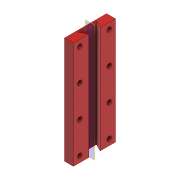
# Autodesk Inventor part: Coupler receiver
Saved by Autodesk Inventor 2020 (Build 240168000, 168)
## iProperties
Created: 2019-11-10
Part Number: Coupler receiver
Material: Generic
Document SubType Name: Modeling
Designer: ball
Density: 1 g/cm^3
Appearance: Default
Author: ball
Autodesk Inventor part; units mm, degrees
ref_plane "YZ Plane" through (0, 0, 0) normal (1, 0, 0) x (0, 1, 0)
ref_plane "XZ Plane" through (0, 0, 0) normal (0, 1, 0) x (-1, 0, 0)
ref_plane "XY Plane" through (0, 0, 0) normal (0, 0, 1) x (1, 0, 0)
sketch "Sketch1" plane through (0, 0, 0) normal (0, 1, 0) x (-1, 0, 0)
  line L0 (0, 17.5) -> (7.366, 17.5)
  line L1 (7.366, 17.5) -> (7.366, -17.5)
  line L2 (7.366, -17.5) -> (0, -17.5)
  line L3 (6.096, 4.754) -> (6.096, -4.754)
  line L4 (0, 4.754) -> (0, 7.802)
  line L5 (6.096, 7.802) -> (6.096, 4.754)
  line L6 (0, -4.754) -> (0, -5.048)
  line L7 (6.096, -7.802) -> (6.096, -4.754)
  line L8 (6.096, 7.802) -> (0, 4.754)
  line L9 (6.096, -7.802) -> (0, -4.754)
  line L10 (0, -17.5) -> (0, -4.754)
  line L11 (0, 4.754) -> (0, 17.5)
  point P0 (0, 0)
  dimension "d0" = 7.366
  dimension "d1" = 35
  dimension "d2" = 17.5
  dimension "d8" = 9.508
  dimension "d9" = 4.754
  dimension "d10" = 3.048
  dimension "d11" = 3.048
  dimension "d12" = 6.096
  dimension "d16" = 15.604
  constraints: 24 end point, 5 parallel, 2 point on line, 1 horizontal, 1 perpendicular
  measures "d0" distance of L1.end L2.end
  measures "d1" distance of L0.end L1.end
  measures "d2" distance from line of L0 point (0, 0)
  measures "d8" distance of L6.start L4.start
  measures "d9" distance of point (0, 0) L4.start
  measures "d10" vertical distance of L5.start L4.start
  measures "d11" vertical distance of L7.start L6.start
  measures "d12" distance from line of L10 L7.start
  measures "d16" distance of L5.start L7.start
extrude "Shape" add sketch "Sketch1" along normal blind 88.9
sketch "Sketch2" plane through (0, 0, -4.754) normal (1, 0, 0) x (0, 0, -1)
  circle A0 centre (7.5184, 5.08) radius 1.9304
  line L0 (3.048, 0) -> (3.048, 88.9) construction
  line L1 (-12.556, 0) -> (-12.556, 88.9) construction
  line L2 (0, 0) -> (12.746, 0) construction
  line L3 (0, 88.9) -> (12.746, 88.9) construction
  circle A1 centre (7.5184, 31.3267) radius 1.9304
  circle A2 centre (7.5184, 57.5733) radius 1.9304
  circle A3 centre (7.5184, 83.82) radius 1.9304
  circle A4 centre (-17.0264, 5.08) radius 1.9304
  line L4 (-22.254, 0) -> (-9.508, 0) construction
  circle A5 centre (-17.0264, 31.3267) radius 1.9304
  circle A6 centre (-17.0264, 57.5733) radius 1.9304
  circle A7 centre (-17.0264, 83.82) radius 1.9304
  point P0 (-4.754, 0)
  dimension "d19" = 3.8608
  dimension "d20" = 4.4704
  dimension "d21" = 88.9
  dimension "d22" = 5.08
  dimension "d25" = 26.2467
  dimension "d30" = 3.8608
  dimension "d31" = 4.4704
  dimension "d32" = 5.08
  dimension "d35" = 26.2467
  constraints: 8 centre point, 2 vertical, 12 other
  measures "d19" diameter of A0
  measures "d20" distance from line of L0 A0.centre
  measures "d21" distance between parallel lines of L2 L3
  measures "d22" distance from line of L2 A0.centre
  measures "d25" distance of A0.centre A1.centre
  measures "d30" diameter of A4
  measures "d31" distance from line of A4.centre L1
  measures "d32" distance from line of L4 A4.centre
  measures "d35" distance of A4.centre A5.centre
extrude "Extrusion2" cut sketch "Sketch2" against normal through all
ref_plane "Work Plane1" through (0, 0, 0) normal (0, 0, -1) x (-1, 0, 0)
equation "\"d2\" = 0.5 * d1"
equation "\"d9\" = 0.5 * d8"
equation "\"d11\" = d10"
equation "\"d31\" = d20"
equation "\"d32\" = d22"
body "Solid1"
